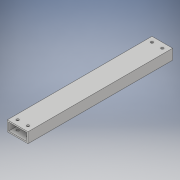
# Autodesk Inventor part: support beam 1
Saved by Autodesk Inventor 2017 (Build 210142000, 142)
## iProperties
Created: 2017-12-29
Part Number: support beam 1
Material: Generic
Document SubType Name: Modeling
Designer: Micah
Density: 1 g/cm^3
Appearance: Default
Author: Micah
Autodesk Inventor part; units mm, degrees
ref_plane "YZ Plane" through (0, 0, 0) normal (1, 0, 0) x (0, 1, 0)
ref_plane "XZ Plane" through (0, 0, 0) normal (0, 1, 0) x (-1, 0, 0)
ref_plane "XY Plane" through (0, 0, 0) normal (0, 0, 1) x (1, 0, 0)
sketch "Sketch1" plane through (0, 0, 0) normal (0, 0, 1) x (1, 0, 0)
  line L0 (0, 0) -> (50.8, 0)
  line L1 (50.8, 0) -> (50.8, 25.4)
  line L2 (50.8, 25.4) -> (0, 25.4)
  line L3 (0, 25.4) -> (0, 0)
  line L4 (3.175, 22.225) -> (47.625, 22.225)
  line L5 (47.625, 22.225) -> (47.625, 3.175)
  line L6 (47.625, 3.175) -> (3.175, 3.175)
  line L7 (3.175, 3.175) -> (3.175, 22.225)
  dimension "d0" = 50.8
  dimension "d1" = 25.4
  dimension "d2" = 44.45
  dimension "d3" = 19.05
  dimension "d4" = 3.175
  dimension "d5" = 3.175
  constraints: 16 end point, 4 parallel, 2 horizontal, 2 perpendicular
  measures "d0" distance of L2.end L1.end
  measures "d1" distance of L1.end L0.end
  measures "d2" distance of L5.end L6.end
  measures "d3" distance of L4.end L5.end
  measures "d4" distance between parallel lines of L2 L4
  measures "d5" distance between parallel lines of L3 L7
extrude "Extrusion1" add sketch "Sketch1" along normal blind 355.6
sketch "Sketch2" plane through (0, 25.4, 0) normal (0, 1, 0) x (1, 0, 0)
  circle A0 centre (12.7, -342.9) radius 3.175
  line L0 (0, -355.6) -> (50.8, -355.6) projected
  line L1 (25.4, -355.6) -> (25.4, 0)
  line L2 (0, 0) -> (0, -355.6) projected
  circle A1 centre (38.1, -342.9) radius 3.175
  line L3 (0, -177.8) -> (50.8, -177.8)
  circle A2 centre (12.7, -12.7) radius 3.175
  circle A3 centre (38.1, -12.7) radius 3.175
  dimension "d8" = 6.35
  dimension "d9" = 12.7
  dimension "d10" = 12.7
  constraints: 4 centre point, 4 end point, 3 symmetric about line, 2 midpoint, 1 horizontal, 1 vertical, 3 other
  measures "d8" diameter of A0
  measures "d9" distance from line of L0 A0.centre
  measures "d10" distance from line of A0.centre L2
hole "Hole1" at (12.7, 25.4, 342.9) at (38.1, 25.4, 342.9) at (12.7, 25.4, 12.7) at (38.1, 25.4, 12.7) direction (0, -1, 0) diameter 6.35 depth 25.4 tip angle 118
body "Solid1"
